# Autodesk Inventor part: JP1B_1X03
Saved by Autodesk Inventor 2016 (Build 200138000, 138)
## iProperties
Created: 2016-04-08
Part Number: JP1B_1X03
Material: Generic
Document SubType Name: Modeling
Designer: Paschalis
Density: 1 g/cm^3
Appearance: 1X03, JP1B_1X03
Author: Paschalis
Autodesk Inventor part; units mm, degrees
ref_plane "YZ Plane" through (0, 0, 0) normal (1, 0, 0) x (0, 1, 0)
ref_plane "XZ Plane" through (0, 0, 0) normal (0, 1, 0) x (-1, 0, 0)
ref_plane "XY Plane" through (0, 0, 0) normal (0, 0, 1) x (1, 0, 0)
sketch "1X03, JP1B_1X03_71" plane through (0, 0, 0) normal (0, 0, 1) x (1, 0, 0)
  line L0 (-1.27, 1.3716) -> (6.35, 1.3716)
  line L1 (6.35, 1.3716) -> (6.35, -1.27)
  line L2 (6.35, -1.27) -> (-1.27, -1.27)
  line L3 (-1.27, -1.27) -> (-1.27, 1.3716)
  constraints: 8 end point
extrude "Extrusion1" add sketch "1X03, JP1B_1X03_71" along normal blind 1
body "Solid1"
